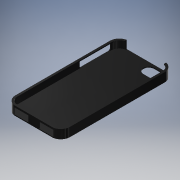
# Autodesk Inventor part: 20150615 IPHONE
Saved by Autodesk Inventor 2019 (Build 230136000, 136)
## iProperties
Created: 2015-06-15
Part Number: 20150615 IPHONE
Material: 일반
Document SubType Name: Modeling
Designer: moon
Density: 1 g/cm^3
Appearance: 기본값
Author: moon
Autodesk Inventor part; units mm, degrees
ref_plane "YZ Plane" through (0, 0, 0) normal (1, 0, 0) x (0, 1, 0)
ref_plane "XZ Plane" through (0, 0, 0) normal (0, 1, 0) x (-1, 0, 0)
ref_plane "XY Plane" through (0, 0, 0) normal (0, 0, 1) x (1, 0, 0)
sketch "스케치1" plane through (0, 0, 0) normal (0, 0, 1) x (1, 0, 0)
  line L0 (-20.2, -62.15) -> (20.2, -62.15)
  line L1 (29.5, -52.85) -> (29.5, 52.85)
  line L2 (20.2, 62.15) -> (-20.2, 62.15)
  line L3 (-29.5, 52.85) -> (-29.5, -52.85)
  line L4 (-29.5, -62.15) -> (29.5, 62.15) construction
  line L5 (29.5, -62.15) -> (-29.5, 62.15) construction
  arc A0 (-20.2, 62.15) -> (-29.5, 52.85) centre (-20.2, 52.85) ccw
  arc A1 (29.5, 52.85) -> (20.2, 62.15) centre (20.2, 52.85) ccw
  arc A2 (20.2, -62.15) -> (29.5, -52.85) centre (20.2, -52.85) ccw
  arc A3 (-29.5, -52.85) -> (-20.2, -62.15) centre (-20.2, -52.85) ccw
  point P0 (0, 0)
  dimension "d0" = 59
  dimension "d1" = 124.3
  dimension "d2" = 9.3
  constraints: 12 end point, 8 point on circle, 8 point on line, 8 tangent, 4 centre point, 3 equal radius, 2 midpoint, 2 parallel, 1 horizontal, 1 perpendicular
  measures "d0" distance of L4.end L5.end
  measures "d1" distance of L5.start L4.end
  measures "d2" radius of A0
extrude "돌출1" add sketch "스케치1" against normal blind 1
sketch "Sketch2" plane through (0, 0, -1) normal (0, 0, -1) x (-1, 0, 0)
  line L0 (29.5, -52.85) -> (29.5, 52.85) projected
  arc A0 (29.5, 52.85) -> (20.2, 62.15) centre (20.2, 52.85) ccw projected
  line L1 (20.2, 62.15) -> (-20.2, 62.15) projected
  arc A1 (-20.2, 62.15) -> (-29.5, 52.85) centre (-20.2, 52.85) ccw projected
  line L2 (-29.5, 52.85) -> (-29.5, -52.85) projected
  arc A2 (-29.5, -52.85) -> (-20.2, -62.15) centre (-20.2, -52.85) ccw projected
  line L3 (-20.2, -62.15) -> (20.2, -62.15) projected
  arc A3 (20.2, -62.15) -> (29.5, -52.85) centre (20.2, -52.85) ccw projected
  point P0 (0, 0)
sketch "스케치3" plane through (0, 0, 0) normal (1, 0, 0) x (0, 1, 0)
  line L0 (62.15, -1) -> (62.15, 7.9)
  line L1 (62.15, 7.9) -> (60.85, 7.9)
  line L2 (60.85, 7.9) -> (60.85, 8.9)
  line L3 (62.15, 0) -> (62.15, -1) projected
  line L4 (62.15, -1) -> (63.15, -1)
  line L5 (62.15, -1) -> (63.15, -1) construction
  line L6 (63.15, -1) -> (63.15, 8.9)
  line L7 (60.85, 8.9) -> (63.15, 8.9)
  point P0 (0, 0)
  dimension "d5" = 8.9
  dimension "d6" = 1.3
  dimension "d7" = 1
  dimension "d45" = 1
  dimension "d46" = 0
  dimension "d47" = 9.9
  dimension "d48" = 90
  dimension "d50" = 2.3
  constraints: 14 end point, 4 perpendicular, 1 collinear, 1 horizontal, 1 vertical
  measures "d5" distance of L0.start L0.end
  measures "d6" distance of L0.end L1.end
  measures "d7" distance of L1.end L2.end
  measures "d45" distance of L0.start L4.end
  measures "d46" distance between parallel lines of L4 L5
  measures "d47" distance of L4.end L6.end
  measures "d48" angle of L6 L4
  measures "d50" distance of L2.end L6.end
sweep "스윕1" add profiles "스케치3" path "Sketch2"
sketch "스케치5" plane through (0, 0, 0) normal (0, 1, 0) x (-1, 0, 0)
  line L0 (-22, 13.1343) -> (22, 13.1343)
  line L1 (22, 13.1343) -> (22, 0)
  line L2 (22, 0) -> (-22, 0)
  line L3 (-22, 0) -> (-22, 13.1343)
  line L4 (-20.2, -1) -> (20.2, -1) projected
  point P0 (0, 0)
  dimension "d12" = 44
  dimension "d13" = 1
  dimension "d14" = 22
  constraints: 8 end point, 2 parallel, 1 horizontal, 1 perpendicular
  measures "d12" distance of L0.start L0.end
  measures "d13" distance between parallel lines of L4 L2
  measures "d14" distance from line of L1 point (0, 0)
extrude "돌출2" cut sketch "스케치5" along normal through all both and the other way through all
sketch "스케치6" plane through (0, 0, 0) normal (0, 0, 1) x (1, 0, 0)
  arc A0 (-22, 61.4639) -> (-29, 52.85) centre (-20.2, 52.85) ccw projected
  arc A1 (29, 52.85) -> (22, 61.4639) centre (20.2, 52.85) ccw projected
  line L0 (-22, 65.5479) -> (22, 65.5479)
  line L1 (22, 65.5479) -> (22, 62.15)
  line L2 (22, 62.15) -> (-22, 62.15)
  line L3 (-22, 62.15) -> (-22, 65.5479)
  line L4 (0, 0) -> (68.1127, 0)
  arc A2 (-29, -52.85) -> (-22, -61.4639) centre (-20.2, -52.85) ccw
  arc A3 (22, -61.4639) -> (29, -52.85) centre (20.2, -52.85) ccw
  line L5 (22, -62.9984) -> (22, -61.4639)
  line L6 (-22, -62.9984) -> (-22, -61.4639)
  line L7 (-22, -65.5479) -> (22, -65.5479)
  line L8 (22, -65.5479) -> (22, -62.15)
  line L9 (22, -62.15) -> (-22, -62.15)
  line L10 (-22, -62.15) -> (-22, -65.5479)
  point P0 (-20.2, -63.1568)
  point P1 (20.2, -63.1568)
  dimension "d17" = 44
  dimension "d18" = 22
  dimension "d19" = 62.15
  constraints: 22 end point, 6 symmetric about line, 4 point on circle, 2 centre point, 2 parallel, 2 perpendicular, 1 horizontal, 2 other
  measures "d17" distance of L0.start L0.end
  measures "d18" distance from line of L3 L4.start
  measures "d19" distance from line of L4.start L2
extrude "돌출3" cut sketch "스케치6" against normal blind 1
sketch "스케치9" plane through (0, 0, -1) normal (0, 0, -1) x (-1, 0, 0)
  line L0 (22, 62.15) -> (-22, 62.15) projected
  line L1 (-19.5, 54.15) -> (-11.5, 54.15) construction
  line L2 (-19.5, 48.15) -> (-11.5, 48.15)
  line L3 (-11.5, 60.15) -> (-19.5, 60.15)
  arc A0 (-19.5, 60.15) -> (-19.5, 48.15) centre (-19.5, 54.15) ccw
  arc A1 (-11.5, 48.15) -> (-11.5, 60.15) centre (-11.5, 54.15) ccw
  point P0 (20.2, 62.15)
  point P1 (-20.2, 62.15)
  point P2 (0, 0)
  point P3 (-15.5, 54.15)
  dimension "d36" = 6
  dimension "d37" = 8
  dimension "d38" = 2
  dimension "d39" = 11.5
  constraints: 8 end point, 4 point on circle, 4 tangent, 2 centre point, 2 parallel, 1 midpoint
  measures "d36" radius of A1
  measures "d37" distance of L1.start L1.end
  measures "d38" distance between parallel lines of L3 L0
  measures "d39" horizontal distance of L1.end point (0, 0)
extrude "돌출6" cut sketch "스케치9" against normal blind 1
sketch "Sketch12" plane through (-30.5, -52.85, -1) normal (-1, 0, 0) x (0, 0, 1)
  line L0 (8.9, 105.7) -> (9.9, 105.7) projected
  line L1 (9.9, 105.7) -> (9.9, 70.7)
  line L2 (9.9, 105.7) -> (9.9, 0) projected
  line L3 (9.9, 105.7) -> (44.9, 105.7) construction
  line L4 (9.9, 70.7) -> (1, 70.7)
  line L5 (1, 0) -> (1, 105.7) projected
  line L6 (1, 70.7) -> (1, 105.7)
  line L7 (1, 105.7) -> (9.9, 105.7)
  line L8 (9.9, 105.7) -> (8.4, 105.7)
  line L9 (9.9, 105.7) -> (9.9, 113.4949) projected
  line L10 (9.9, 105.7) -> (11.4, 105.7) construction
  line L11 (8.4, 105.7) -> (8.4, 70.7)
  line L12 (8.4, 105.7) -> (1, 105.7)
  line L13 (1, 105.7) -> (1, 70.7)
  line L14 (1, 70.7) -> (8.4, 70.7)
  line L15 (8.4, 70.7) -> (8.4, 105.7)
  point P0 (1, 52.85)
  dimension "d51" = 35
  dimension "d52" = 90
  dimension "d53" = 8.9
  dimension "d54" = 90
  dimension "d55" = 35
  dimension "d56" = 90
  dimension "d57" = 8.9
  dimension "d58" = 90
  dimension "d59" = 1.5
  dimension "d60" = 180
  dimension "d61" = 35
  dimension "d62" = 90
  dimension "d63" = 7.4
  dimension "d64" = 35
  constraints: 24 end point, 4 perpendicular, 3 horizontal, 2 equal length, 2 parallel, 1 collinear
  measures "d51" distance of L0.end L1.end
  measures "d52" angle of L1 L3
  measures "d53" distance of L1.end L4.end
  measures "d54" angle of L1 L4
  measures "d55" distance of L4.end L5.end
  measures "d56" angle of L4 L6
  measures "d57" distance of L5.end L0.end
  measures "d58" angle of L6 L7
  measures "d59" distance of L0.end L8.end
  measures "d60" angle of L8 L10
  measures "d61" distance of L8.end L11.end
  measures "d62" angle of L11 L8
  measures "d63" distance of L14.end L4.end
  measures "d64" distance of L4.end L12.end
extrude "Extrusion8" cut sketch "Sketch12" against normal blind 10 contours L11 L4 L5 L7
fillet "Fillet8" radius 2 4 edges at (-30, 17.85, 7.4) (-30, 17.85, 0) (-30, 52.85, 0) (-30, 52.85, 7.4)
sketch "Sketch13" plane through (-22, -62.15, 0) normal (0, -1, 0) x (1, 0, 0)
  line L0 (52.5, -1) -> (44, -1) projected
  line L1 (0, 0) -> (44, 0) projected
  line L2 (44, -1) -> (0, -1)
  line L3 (0, -1) -> (0, 0)
  line L4 (0, 0) -> (44, 0)
  line L5 (44, 0) -> (44, -1)
  point P0 (22, 0)
  dimension "d68" = 44
  dimension "d69" = 1
  constraints: 8 end point, 2 parallel, 1 horizontal, 1 perpendicular
  measures "d68" distance of L1.start L4.end
  measures "d69" distance of L2.end L1.start
extrude "Extrusion9" add sketch "Sketch13" along normal blind 0.8415
sketch "Sketch14" plane through (-22, 62.15, 0) normal (0, 1, 0) x (1, 0, 0)
  line L0 (0, 1) -> (0, 0) projected
  line L1 (0, 1) -> (44, 1)
  line L2 (44, 1) -> (44, 0)
  line L3 (44, 0) -> (0, 0)
  line L4 (0, 0) -> (0, 1)
  point P0 (22, 0)
  dimension "d72" = 44
  dimension "d73" = 1
  constraints: 8 end point, 2 parallel, 1 horizontal, 1 perpendicular
  measures "d72" distance of L2.end L3.end
  measures "d73" distance of L1.end L2.end
extrude "Extrusion10" add sketch "Sketch14" along normal blind 0.8415
sketch "Sketch15" plane through (0, 0, 0) normal (0, 0, 1) x (1, 0, 0)
  arc A0 (22, -62.9915) -> (30.5, -52.85) centre (20.2, -52.85) ccw projected
  line L0 (22, -62.9915) -> (0, -62.9915)
  line L1 (22, -62.9915) -> (-22, -62.9915) projected
  line L2 (22, -62.9915) -> (44, -62.9915) construction
  line L3 (0, -62.9915) -> (6, -62.9915)
  line L4 (6, -62.9915) -> (6, -61.9915)
  line L5 (6, -61.9915) -> (0, -61.9915)
  line L6 (0, -61.9915) -> (0, -62.9915)
  line L7 (0, -62.9915) -> (-6, -62.9915)
  line L8 (-6, -62.9915) -> (-6, -61.9915)
  line L9 (-6, -61.9915) -> (0, -61.9915)
  line L10 (0, -61.9915) -> (0, -62.9915)
  point P0 (0, 0)
  dimension "d76" = 22
  dimension "d77" = 180
  dimension "d78" = 6
  dimension "d79" = 1
  dimension "d80" = 6
  dimension "d81" = 1
  constraints: 20 end point, 5 parallel, 3 horizontal, 2 perpendicular, 1 collinear
  measures "d76" distance of L0.start L0.end
  measures "d77" angle of L2 L0
  measures "d78" distance of L5.end L4.end
  measures "d79" distance of L4.end L3.end
  measures "d80" distance of L8.end L9.end
  measures "d81" distance of L7.end L8.end
extrude "Extrusion11" add sketch "Sketch15" along normal blind 8.9
sketch "Sketch16" plane through (22, -62.9915, 8.9) normal (-1, 0, 0) x (0, 0, 1)
  line L0 (0, 0) -> (-1, 0)
  line L1 (-1, 0) -> (-1, 2.347)
  line L2 (-1, 2.347) -> (0, 2.347)
  line L3 (0, 2.347) -> (0, 0)
  line L4 (-1, 0) -> (-2, 0)
  line L5 (-2, 0) -> (-2, 1.017)
  line L6 (-2, 1.017) -> (-1, 1.017)
  line L7 (-1, 1.017) -> (-1, 0)
  point P0 (-8.9, 62.9915)
  dimension "d84" = 1
  dimension "d85" = 2.347
  dimension "d88" = 1
  dimension "d89" = 1.017
  constraints: 16 end point, 4 parallel, 2 horizontal, 2 perpendicular
  measures "d84" distance of L1.end L2.end
  measures "d85" distance of L0.end L1.end
  measures "d88" distance of L5.end L6.end
  measures "d89" distance of L4.end L5.end
extrude "Extrusion12" add sketch "Sketch16" along normal blind 44
sketch "Sketch17" plane through (0, 0, -1) normal (0, 0, -1) x (-1, 0, 0)
  line L0 (22, -62.9915) -> (-22, -62.9915) projected
  line L1 (0, -62.9915) -> (0, -41.9915)
  line L2 (0, -62.9915) -> (21, -62.9915) construction
  line L3 (0, -41.9915) -> (-0.5, -41.9915)
  line L4 (-0.5, -41.9915) -> (-0.5, 43.0085)
  line L5 (-0.5, 43.0085) -> (0, 43.0085)
  line L6 (0, 43.0085) -> (0, -41.9915)
  line L7 (0, 43.0085) -> (0.5, 43.0085)
  line L8 (0.5, 43.0085) -> (0.5, -41.9915)
  line L9 (0.5, -41.9915) -> (0, -41.9915)
  line L10 (0, -41.9915) -> (0, 43.0085)
  point P0 (0, 0)
  dimension "d90" = 21
  dimension "d91" = 90
  dimension "d92" = 0.5
  dimension "d93" = 85
  dimension "d94" = 0.5
  dimension "d95" = 85
  constraints: 20 end point, 4 parallel, 3 horizontal, 3 perpendicular, 1 midpoint, 1 vertical
  measures "d90" distance of L1.start L1.end
  measures "d91" angle of L2 L1
  measures "d92" distance of L4.end L5.end
  measures "d93" distance of L3.end L4.end
  measures "d94" distance of L8.end L9.end
  measures "d95" distance of L7.end L8.end
extrude "Extrusion13" add sketch "Sketch17" along normal blind 2.1
sketch "Sketch18" plane through (0.5, -41.9915, -1) normal (1, 0, 0) x (0, 0, -1)
  line L0 (2.1, 85) -> (2.1, 0) projected
  line L1 (2.1, 0) -> (1.1, 0)
  line L2 (1.1, 0) -> (1.1, 85)
  line L3 (1.1, 85) -> (2.1, 85)
  line L4 (2.1, 85) -> (2.1, 0)
  point P0 (-1, 41.9915)
  dimension "d98" = 1
  dimension "d99" = 85
  constraints: 8 end point, 2 parallel, 1 horizontal, 1 perpendicular
  measures "d98" distance of L2.end L3.end
  measures "d99" distance of L1.end L2.end
extrude "Extrusion14" add sketch "Sketch18" along normal blind 1.1 and the other way blind 2.1
sketch "Sketch19" plane through (0, 0, -1) normal (0, 0, -1) x (-1, 0, 0)
  line L0 (-0.5, -41.9915) -> (-0.5, 43.0085) projected
  line L1 (-0.5, -41.9915) -> (-25.2, -41.9915)
  line L2 (-0.5, -41.9915) -> (24.2, -41.9915) construction
  line L3 (-25.2, -41.9915) -> (-26.2, -41.9915)
  line L4 (-26.2, -41.9915) -> (-26.2, 43.0085)
  line L5 (-26.2, 43.0085) -> (-25.2, 43.0085)
  line L6 (-25.2, 43.0085) -> (-25.2, -41.9915)
  line L7 (0.5, 43.0085) -> (0.5, -41.9915) projected
  line L8 (0.5, -41.9915) -> (25.2, -41.9915)
  line L9 (0.5, -41.9915) -> (25.2, -41.9915) construction
  line L10 (25.2, -41.9915) -> (26.2, -41.9915)
  line L11 (26.2, -41.9915) -> (26.2, 43.0085)
  line L12 (26.2, 43.0085) -> (25.2, 43.0085)
  line L13 (25.2, 43.0085) -> (25.2, -41.9915)
  point P0 (0, 0)
  dimension "d104" = 24.7
  dimension "d105" = 180
  dimension "d106" = 1
  dimension "d107" = 85
  dimension "d108" = 24.7
  dimension "d109" = 0
  dimension "d110" = 1
  dimension "d111" = 85
  constraints: 24 end point, 5 equal length, 5 horizontal, 2 collinear, 2 perpendicular
  measures "d104" distance of L0.start L1.end
  measures "d105" angle of L1 L2
  measures "d106" distance of L4.end L5.end
  measures "d107" distance of L3.end L4.end
  measures "d108" distance of L7.end L8.end
  measures "d109" distance between parallel lines of L8 L9
  measures "d110" distance of L12.end L11.end
  measures "d111" distance of L11.end L10.end
extrude "Extrusion15" add sketch "Sketch19" along normal blind 2.1
sketch "Sketch20" plane through (25.2, -41.9915, -1) normal (-1, 0, 0) x (0, 0, 1)
  line L0 (-2.1, 0) -> (-2.1, 85) projected
  line L1 (-2.1, 0) -> (-1.1, 0)
  line L2 (-1.1, 0) -> (-1.1, 85)
  line L3 (-1.1, 85) -> (-2.1, 85)
  line L4 (-2.1, 85) -> (-2.1, 0)
  point P0 (1, 41.9915)
  dimension "d114" = 1
  dimension "d115" = 85
  constraints: 8 end point, 2 parallel, 1 horizontal, 1 perpendicular
  measures "d114" distance of L3.end L2.end
  measures "d115" distance of L2.end L1.end
extrude "Extrusion16" add sketch "Sketch20" along normal blind 1
sketch "Sketch21" plane through (-25.2, -41.9915, -1) normal (1, 0, 0) x (0, 0, -1)
  line L0 (0, 0) -> (2.1, 0) projected
  line L1 (2.1, 0) -> (1.1, 0)
  line L2 (1.1, 0) -> (1.1, 85)
  line L3 (1.1, 85) -> (2.1, 85)
  line L4 (2.1, 85) -> (2.1, 0)
  point P0 (-1, 41.9915)
  dimension "d118" = 1
  dimension "d119" = 85
  constraints: 8 end point, 2 parallel, 1 horizontal, 1 perpendicular
  measures "d118" distance of L2.end L3.end
  measures "d119" distance of L1.end L2.end
extrude "Extrusion17" add sketch "Sketch21" along normal blind 1
